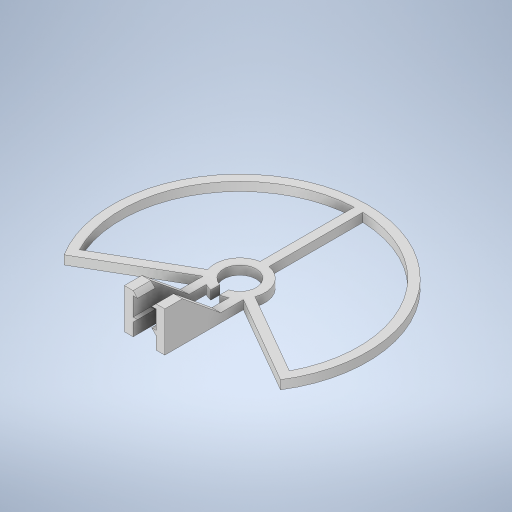
# Autodesk Inventor part: ProtectorHelice
Saved by Autodesk Inventor 2024.3 (Build 283343000, 343)
## iProperties
Created: 2024-10-09
Part Number: ProtectorHelice
Material: Generic
Document SubType Name: Modeling
Designer: pjcaa
Density: 1 g/cm^3
Appearance: Default
Author: pjcaa
Autodesk Inventor part; units mm, degrees
ref_plane "YZ Plane" through (0, 0, 0) normal (1, 0, 0) x (0, 1, 0)
ref_plane "XZ Plane" through (0, 0, 0) normal (0, 1, 0) x (-1, 0, 0)
ref_plane "XY Plane" through (0, 0, 0) normal (0, 0, 1) x (1, 0, 0)
sketch "Sketch1" plane through (0, 0, 0) normal (0, 0, 1) x (1, 0, 0)
  circle A0 centre (0, 0) radius 3.7
  circle A1 centre (0, 0) radius 5.7
  dimension "d0" = 7.4
  dimension "d1" = 11.4
  constraints: 2 centre point, 2 coincident
  measures "d0" diameter of A0
  measures "d1" diameter of A1
extrude "Extrusion1" add sketch "Sketch1" along normal blind 2
sketch "Sketch2" plane through (0, 0, 0) normal (0, 0, 1) x (1, 0, 0)
  circle A0 centre (0, 0) radius 29
  circle A1 centre (0, 0) radius 27
  dimension "d4" = 58
  dimension "d5" = 54
  constraints: 2 centre point, 2 coincident
  measures "d4" diameter of A0
  measures "d5" diameter of A1
extrude "Extrusion2" add sketch "Sketch2" along normal blind 2
sketch "Sketch3" plane through (0, 0, 0) normal (0, 0, 1) x (1, 0, 0)
  line L0 (0, 0) -> (27, 0) construction
  circle A0 centre (0, 0) radius 5.7 construction
  circle A1 centre (0, 0) radius 27 construction
  line L1 (5.6116, 1) -> (26.9815, 1)
  line L2 (26.9815, -1) -> (5.6116, -1)
  arc A2 (5.6116, -1) -> (5.6116, 1) centre (0, 0) ccw
  arc A3 (26.9815, -1) -> (26.9815, 1) centre (0, 0) ccw
  line L3 (-3.6718, 4.3598) -> (-14.3568, 22.8666)
  line L4 (-12.6247, 23.8666) -> (-1.9398, 5.3598)
  arc A4 (-1.9398, 5.3598) -> (-3.6718, 4.3598) centre (0, 0) ccw
  arc A5 (-12.6247, 23.8666) -> (-14.3568, 22.8666) centre (0, 0) ccw
  line L5 (-1.9398, -5.3598) -> (-12.6247, -23.8666)
  line L6 (-14.3568, -22.8666) -> (-3.6718, -4.3598)
  arc A6 (-3.6718, -4.3598) -> (-1.9398, -5.3598) centre (0, 0) ccw
  arc A7 (-14.3568, -22.8666) -> (-12.6247, -23.8666) centre (0, 0) ccw
  dimension "d9" = 11.4
  dimension "d10" = 54
  dimension "d12" = 1
  dimension "d15" = 360
  constraints: 17 point on circle, 14 end point, 8 centre point, 5 coincident, 2 parallel, 2 vertical alignment, 1 horizontal, 31 other
  measures "d9" diameter of A0
  measures "d10" diameter of A1
  measures "d12" vertical distance of point (0, 0) L2.end
extrude "Extrusion3" add sketch "Sketch3" along normal blind 2
sketch "Sketch4" plane through (0, 0, 0) normal (0, 0, 1) x (1, 0, 0)
  arc A0 (5.6116, 1) -> (-1.9398, 5.3598) centre (0, 0) ccw construction
  line L0 (-1.9398, 5.3598) -> (-12.6247, 23.8666) construction
  arc A1 (26.9815, 1) -> (-12.6247, 23.8666) centre (0, 0) ccw construction
  line L1 (26.9815, 1) -> (5.6116, 1) construction
  line L2 (5.6116, -1) -> (26.9815, -1) construction
  arc A2 (-12.6247, -23.8666) -> (26.9815, -1) centre (0, 0) ccw construction
  line L3 (-12.6247, -23.8666) -> (-1.9398, -5.3598) construction
  arc A3 (-1.9398, -5.3598) -> (5.6116, -1) centre (0, 0) ccw construction
  circle A4 centre (0, 0) radius 29 construction
  line L4 (-3.6718, -4.3598) -> (-14.3568, -22.8666) construction
  arc A5 (-14.3568, 22.8666) -> (-14.3568, -22.8666) centre (0, 0) ccw construction
  line L5 (-14.3568, 22.8666) -> (-3.6718, 4.3598) construction
  arc A6 (-3.6718, 4.3598) -> (-3.6718, -4.3598) centre (0, 0) ccw construction
  circle A7 centre (0, 0) radius 3.7 construction
  circle A8 centre (0, 0) radius 29 construction
  arc A9 (-14.3568, 22.8666) -> (-14.3568, -22.8666) centre (0, 0) ccw construction
  line L6 (-14.3568, 22.8666) -> (-15.3574, 24.5998)
  line L7 (-14.3568, -22.8666) -> (-15.3574, -24.5998)
  arc A10 (-15.3574, 24.5998) -> (-15.3574, -24.5998) centre (0, 0) ccw
  arc A11 (-14.3568, 22.8666) -> (-14.3568, -22.8666) centre (0, 0) ccw
  constraints: 6 point on circle, 4 end point, 2 centre point, 1 coincident, 1 collinear, 1 concentric, 1 equal length
extrude "Extrusion4" cut sketch "Sketch4" along normal through all
sketch "Sketch5" plane through (0, 0, 0) normal (0, 0, 1) x (1, 0, 0)
  arc A0 (-3.6718, 4.3598) -> (-3.6718, -4.3598) centre (0, 0) ccw construction
  circle A1 centre (0, 0) radius 3.7 construction
  line L0 (-5.6116, 1) -> (-3.5623, 1)
  line L1 (-3.5623, -1) -> (-5.6116, -1)
  arc A2 (-5.6116, 1) -> (-5.6116, -1) centre (0, 0) ccw
  arc A3 (-3.5623, 1) -> (-3.5623, -1) centre (0, 0) ccw
  dimension "d21" = 1
  constraints: 8 point on circle, 4 end point, 2 centre point, 2 concentric, 2 parallel, 1 horizontal
  measures "d21" distance from line of point (0, 0) L1
extrude "Extrusion5" cut sketch "Sketch5" along normal through all
sketch "Sketch6" plane through (0, 0, 0) normal (0, 0, 1) x (1, 0, 0)
  line L0 (5.6116, -1) -> (26.9815, -1) construction
  arc A0 (-12.6247, -23.8666) -> (26.9815, -1) centre (0, 0) ccw construction
  line L1 (-12.6247, -23.8666) -> (-1.9398, -5.3598) construction
  arc A1 (-1.9398, -5.3598) -> (5.6116, -1) centre (0, 0) ccw construction
  arc A2 (5.6116, 1) -> (-1.9398, 5.3598) centre (0, 0) ccw construction
  line L2 (-1.9398, 5.3598) -> (-12.6247, 23.8666) construction
  arc A3 (26.9815, 1) -> (-12.6247, 23.8666) centre (0, 0) ccw construction
  line L3 (26.9815, 1) -> (5.6116, 1) construction
  line L4 (-3.5623, -1) -> (-5.6116, -1) construction
  arc A4 (-5.6116, -1) -> (-3.6718, -4.3598) centre (0, 0) ccw construction
  line L5 (-3.6718, -4.3598) -> (-15.3574, -24.5998) construction
  arc A5 (-15.3574, -24.5998) -> (-15.3574, 24.5998) centre (0, 0) ccw construction
  line L6 (-15.3574, 24.5998) -> (-3.6718, 4.3598) construction
  arc A6 (-3.6718, 4.3598) -> (-5.6116, 1) centre (0, 0) ccw construction
  line L7 (-5.6116, 1) -> (-3.5623, 1) construction
  arc A7 (-3.5623, -1) -> (-3.5623, 1) centre (0, 0) ccw construction
  line L8 (-5.0725, 2.6) -> (-21.6725, 2.6)
  line L9 (-5.0725, -2.6) -> (-21.6725, -2.6)
  line L10 (-21.6725, 4.6) -> (-3.8105, 4.6)
  line L11 (-21.6725, -4.6) -> (-3.8105, -4.6)
  line L12 (-5.0725, 2.6) -> (-5.0725, -2.6) construction
  line L13 (-3.8105, 4.6) -> (-3.6718, 4.3598)
  line L14 (-3.8105, -4.6) -> (-3.6718, -4.3598)
  arc A8 (-3.6718, 4.3598) -> (-5.0725, 2.6) centre (0, 0) ccw
  arc A9 (-5.0725, -2.6) -> (-3.6718, -4.3598) centre (0, 0) ccw
  line L15 (-21.6725, 4.6) -> (-21.6725, 2.6)
  line L16 (-21.6725, -2.6) -> (-21.6725, -4.6)
  point P0 (-5.0725, 0)
  dimension "d24" = 5.2
  dimension "d25" = 2
  dimension "d26" = 2
  dimension "d27" = 16.6
  constraints: 18 end point, 6 point on circle, 4 horizontal, 3 point on line, 3 vertical alignment, 2 centre point, 2 collinear, 2 concentric, 2 parallel, 2 vertical, 1 horizontal alignment, 1 midpoint
  measures "d24" distance between parallel lines of L9 L8
  measures "d25" distance between parallel lines of L11 L9
  measures "d26" distance between parallel lines of L8 L10
  measures "d27" horizontal distance of L9.start L11.start
extrude "Extrusion6" add sketch "Sketch6" along normal blind 2
sketch "Sketch7" plane through (0, 0, 2) normal (0, 0, 1) x (1, 0, 0)
  line L0 (5.6116, -1) -> (26.9815, -1) construction
  arc A0 (-12.6247, -23.8666) -> (26.9815, -1) centre (0, 0) ccw construction
  line L1 (-12.6247, -23.8666) -> (-1.9398, -5.3598) construction
  arc A1 (-1.9398, -5.3598) -> (5.6116, -1) centre (0, 0) ccw construction
  arc A2 (5.6116, 1) -> (-1.9398, 5.3598) centre (0, 0) ccw construction
  line L2 (-1.9398, 5.3598) -> (-12.6247, 23.8666) construction
  arc A3 (26.9815, 1) -> (-12.6247, 23.8666) centre (0, 0) ccw construction
  line L3 (26.9815, 1) -> (5.6116, 1) construction
  line L4 (-3.5623, -1) -> (-5.6116, -1) construction
  arc A4 (-5.6116, -1) -> (-5.0725, -2.6) centre (0, 0) ccw construction
  line L5 (-5.0725, -2.6) -> (-21.6725, -2.6) construction
  line L6 (-21.6725, -2.6) -> (-21.6725, -4.6) construction
  line L7 (-21.6725, -4.6) -> (-3.8105, -4.6) construction
  line L8 (-3.8105, -4.6) -> (-15.3574, -24.5998) construction
  arc A5 (-15.3574, -24.5998) -> (-15.3574, 24.5998) centre (0, 0) ccw construction
  line L9 (-15.3574, 24.5998) -> (-3.8105, 4.6) construction
  line L10 (-3.8105, 4.6) -> (-21.6725, 4.6) construction
  line L11 (-21.6725, 4.6) -> (-21.6725, 2.6) construction
  line L12 (-21.6725, 2.6) -> (-5.0725, 2.6) construction
  arc A6 (-5.0725, 2.6) -> (-5.6116, 1) centre (0, 0) ccw construction
  line L13 (-5.6116, 1) -> (-3.5623, 1) construction
  arc A7 (-3.5623, -1) -> (-3.5623, 1) centre (0, 0) ccw construction
  line L14 (-21.6725, 4.6) -> (-17.6725, 4.6)
  line L15 (-17.6725, 4.6) -> (-17.6725, 2.6)
  line L16 (-17.6725, 2.6) -> (-21.6725, 2.6)
  line L17 (-21.6725, 2.6) -> (-21.6725, 4.6)
  line L18 (-21.6725, -2.6) -> (-17.6725, -2.6)
  line L19 (-17.6725, -2.6) -> (-17.6725, -4.6)
  line L20 (-17.6725, -4.6) -> (-21.6725, -4.6)
  line L21 (-21.6725, -4.6) -> (-21.6725, -2.6)
  dimension "d30" = 4
  dimension "d31" = 4
  constraints: 16 end point, 4 parallel, 2 horizontal, 2 perpendicular, 2 point on line
  measures "d30" distance of L15.end L16.end
  measures "d31" distance of L19.end L20.end
extrude "Extrusion7" add sketch "Sketch7" along normal blind 7.1
chamfer "Chamfer1" distance 8.7 distance2 7.1 2 edges at (-17.6725, -3.6, 2) (-17.6725, 3.6, 2) measured on face at (-17.1725, 3.6, 2) measured on face at (-17.1725, -3.6, 2)
sketch "Sketch8" plane through (-21.6725, 2.6, 0) normal (-1, 0, 0) x (0, 0, 1)
  line L0 (0, -5.2) -> (9.1, -5.2) construction
  line L1 (0, 0) -> (9.1, 0) construction
  line L2 (9.1, 0) -> (8.1, -1)
  line L3 (8.1, -1) -> (8.1, 0)
  line L4 (8.1, 0) -> (9.1, 0)
  line L5 (2.9, 0) -> (3.9, 0)
  line L6 (3.9, -1) -> (3.9, 0)
  line L7 (3.9, -1) -> (2.9, 0)
  line L8 (9.1, -5.2) -> (9.1, 0) construction
  line L9 (0, -2.6) -> (9.1, -2.6) construction
  line L10 (9.1, -5.2) -> (8.1, -4.2)
  line L11 (8.1, -4.2) -> (8.1, -5.2)
  line L12 (8.1, -5.2) -> (9.1, -5.2)
  line L13 (2.9, -5.2) -> (3.9, -5.2)
  line L14 (3.9, -4.2) -> (3.9, -5.2)
  line L15 (3.9, -4.2) -> (2.9, -5.2)
  dimension "d37" = 1
  dimension "d38" = 1
  dimension "d39" = 4.2
  constraints: 28 end point, 6 symmetric about line, 3 perpendicular, 3 point on line, 1 collinear, 1 horizontal, 1 horizontal alignment, 1 midpoint, 1 vertical
  measures "d37" distance of L2.end L3.end
  measures "d38" distance from line of L1.end L3
  measures "d39" distance between parallel lines of L3 L6
extrude "Extrusion8" add sketch "Sketch8" against normal blind 4
body "Solid1"
